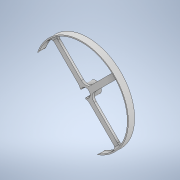
# Autodesk Inventor part: GuardV2
Saved by Autodesk Inventor 2020 (Build 240168000, 168)
## iProperties
Created: 2023-01-16
Part Number: GuardV2
Material: Generic
Document SubType Name: Modeling
Designer: agraa4529
Density: 1 g/cm^3
Appearance: Default
Author: agraa4529
## iProperties of the stored document _3DPrint.ipt
Created: 2023-01-16
Part Number: _3DPrint
Material: Generic
Document SubType Name: Modeling
Designer: agraa4529
Density: 1 g/cm^3
Appearance: Default
Author: agraa4529
Autodesk Inventor part; units mm, degrees
ref_plane "YZ Plane" through (0, 0, 0) normal (1, 0, 0) x (0, 1, 0)
ref_plane "XZ Plane" through (0, 0, 0) normal (0, 1, 0) x (-1, 0, 0)
ref_plane "XY Plane" through (0, 0, 0) normal (0, 0, 1) x (1, 0, 0)
sketch "Sketch1" plane through (0, 0, 0) normal (0, 0, 1) x (1, 0, 0)
  arc A0 (0, -4.125) -> (-4.0608, 0.7248) centre (0, 0) ccw
  line L0 (0, -4.125) -> (-4.0608, 0.7248)
  arc A1 (-0.4919, -5.3424) -> (-5.3588, 0.2578) centre (0, 0) ccw
  line L1 (0, -4.125) -> (-0.4919, -5.3424)
  line L2 (0, -4.125) -> (1.313, -4.125) construction
  line L3 (-4.0608, 0.7248) -> (-5.3588, 0.2578)
  dimension "d0" = 8.25
  dimension "d1" = 10.73
  dimension "d2" = 112
  constraints: 8 end point, 4 point on circle, 2 centre point, 2 coincident, 1 equal length, 1 horizontal
  measures "d0" diameter of A0
  measures "d1" diameter of A1
  measures "d2" angle of L1 L2
extrude "Extrusion1" add sketch "Sketch1" along normal blind 9.5 contours A0 L3 A1 L1
sketch "Sketch2" plane through (0, 0, 9.5) normal (0, 0, 1) x (1, 0, 0)
  arc A0 (-0.4919, -5.3424) -> (-5.3588, 0.2578) centre (0, 0) ccw projected
  line L0 (0, 5.365) -> (5.365, 0) construction
  line L1 (3.7936, 3.7936) -> (0, 5.365) construction
  line L2 (3.7936, 3.7936) -> (5.365, 0) construction
  line L3 (3.7936, 3.7936) -> (5.5269, 2.0604)
  line L4 (5.5269, 2.0604) -> (32.5269, 29.0604)
  line L5 (32.5269, 29.0604) -> (30.7936, 30.7936)
  line L6 (30.7936, 30.7936) -> (3.7936, 3.7936)
  line L7 (1.9965, 5.5907) -> (28.9965, 32.5907)
  line L8 (28.9965, 32.5907) -> (30.7936, 30.7936)
  line L9 (1.9965, 5.5907) -> (3.7936, 3.7936)
  line L10 (1.9965, 5.5907) -> (5.5269, 2.0604)
  line L11 (5.5269, 2.0604) -> (4.7391, 1.2726)
  line L12 (4.7391, 1.2726) -> (1.2088, 4.8029)
  line L13 (1.2088, 4.8029) -> (1.9965, 5.5907)
  line L14 (-3.7936, 3.7936) -> (-5.365, 0) construction
  line L15 (-3.7936, 3.7936) -> (-2.0604, 5.5269)
  line L16 (-2.0604, 5.5269) -> (-29.0604, 32.5269)
  line L17 (-29.0604, 32.5269) -> (-30.7936, 30.7936)
  line L18 (-30.7936, 30.7936) -> (-3.7936, 3.7936)
  line L19 (-5.5907, 1.9965) -> (-32.5907, 28.9965)
  line L20 (-32.5907, 28.9965) -> (-30.7936, 30.7936)
  line L21 (-5.5907, 1.9965) -> (-3.7936, 3.7936)
  line L22 (-5.5907, 1.9965) -> (-2.0604, 5.5269)
  line L23 (-2.0604, 5.5269) -> (-1.2726, 4.7391)
  line L24 (-1.2726, 4.7391) -> (-4.8029, 1.2088)
  line L25 (-4.8029, 1.2088) -> (-5.5907, 1.9965)
  line L26 (-3.7936, -3.7936) -> (0, -5.365) construction
  line L27 (-3.7936, -3.7936) -> (-5.5269, -2.0604)
  line L28 (-5.5269, -2.0604) -> (-32.5269, -29.0604)
  line L29 (-32.5269, -29.0604) -> (-30.7936, -30.7936)
  line L30 (-30.7936, -30.7936) -> (-3.7936, -3.7936)
  line L31 (-1.9965, -5.5907) -> (-28.9965, -32.5907)
  line L32 (-28.9965, -32.5907) -> (-30.7936, -30.7936)
  line L33 (-1.9965, -5.5907) -> (-3.7936, -3.7936)
  line L34 (-1.9965, -5.5907) -> (-5.5269, -2.0604)
  line L35 (-5.5269, -2.0604) -> (-4.7391, -1.2726)
  line L36 (-4.7391, -1.2726) -> (-1.2088, -4.8029)
  line L37 (-1.2088, -4.8029) -> (-1.9965, -5.5907)
  line L38 (3.7936, -3.7936) -> (5.365, 0) construction
  line L39 (3.7936, -3.7936) -> (2.0604, -5.5269)
  line L40 (2.0604, -5.5269) -> (29.0604, -32.5269)
  line L41 (29.0604, -32.5269) -> (30.7936, -30.7936)
  line L42 (30.7936, -30.7936) -> (3.7936, -3.7936)
  line L43 (5.5907, -1.9965) -> (32.5907, -28.9965)
  line L44 (32.5907, -28.9965) -> (30.7936, -30.7936)
  line L45 (5.5907, -1.9965) -> (3.7936, -3.7936)
  line L46 (5.5907, -1.9965) -> (2.0604, -5.5269)
  line L47 (2.0604, -5.5269) -> (1.2726, -4.7391)
  line L48 (1.2726, -4.7391) -> (4.8029, -1.2088)
  line L49 (4.8029, -1.2088) -> (5.5907, -1.9965)
  dimension "d5" = 27
  dimension "d6" = 27
  dimension "d11" = 360
  constraints: 100 end point, 4 parallel, 3 point on circle, 2 coincident, 2 collinear, 2 perpendicular, 2 tangent, 91 other
  measures "d5" horizontal distance of L5.end L1.start
  measures "d6" horizontal distance of L5.end L1.start
extrude "Extrusion2" add sketch "Sketch2" against normal blind 2 contours L47 L48 L49 A0 | A0 L39 L47 | L42 L41 L40 L39 | L45 L43 L44 L42 | A0 L49 L45 | L11 L12 L13 A0 | A0 L3 L11 | L6 L5 L4 L3 | L9 L7 L8 L6 | A0 L13 L9 | L23 L24 L25 A0 | A0 L15 L23 | L18 L17 L16 L15 | L21 L19 L20 L18 | A0 L25 L21
sketch "Sketch3" plane through (0, 0, 9.5) normal (0, 0, 1) x (1, 0, 0)
  circle A0 centre (0, 0) radius 43.5
  circle A1 centre (0, 0) radius 44.5
  dimension "d13" = 87
  dimension "d14" = 89
  constraints: 2 centre point, 2 coincident
  measures "d13" diameter of A0
  measures "d14" diameter of A1
extrude "Extrusion3" add sketch "Sketch3" along normal blind 4 and the other way blind 2
fillet "Fillet1" radius 6 2 edges at (1.6413, -5.1078, 8.5) (-5.1381, 1.5439, 8.5)
fillet "Fillet2" radius 6 4 edges at (-1.6413, 5.1078, 8.5) (1.5439, 5.1381, 8.5) (5.1078, 1.6413, 8.5) (5.1381, -1.5439, 8.5)
fillet "Fillet3" radius 2 3 edges at (30.7272, 30.7911, 9.5) (-30.7911, 30.7272, 9.5) (30.7911, -30.7272, 9.5)
fillet "Fillet4" radius 3 12 edges at (32.4435, 28.977, 10.5) (32.4435, 28.977, 8.5) (28.9095, 32.5037, 10.5) (28.9095, 32.5037, 8.5) (-28.977, 32.4435, 10.5) (-28.977, 32.4435, 8.5) (-32.5037, 28.9095, 10.5) (-32.5037, 28.9095, 8.5) (28.977, -32.4435, 10.5) (28.977, -32.4435, 8.5) (32.5037, -28.9095, 10.5) (32.5037, -28.9095, 8.5)
sketch "Sketch5" plane through (0, 0, 13.5) normal (0, 0, 1) x (1, 0, 0)
  line L0 (0, 0) -> (-14.1421, -14.1421)
  line L1 (0, 0) -> (20, 0) construction
  line L2 (-14.1421, -14.1421) -> (-52.7132, 24.4289)
  line L3 (-52.7132, 24.4289) -> (-46.2577, -44.0894)
  line L4 (-46.2577, -44.0894) -> (25.7102, -52.0399)
  line L5 (25.7102, -52.0399) -> (-14.1421, -14.1421)
  dimension "d23" = 20
  dimension "d24" = 135
  dimension "d25" = 90
  constraints: 12 end point, 1 equal length, 1 horizontal
  measures "d23" distance of L0.start L0.end
  measures "d24" angle of L0 L1
  measures "d25" angle of L0 L2
extrude "Extrusion4" cut sketch "Sketch5" against normal blind 9.5
fillet "Fillet5" radius 4 2 edges at (-41.4574, 13.1732, 10.5) (14.2176, -41.111, 10.5)
body "Solid1"
